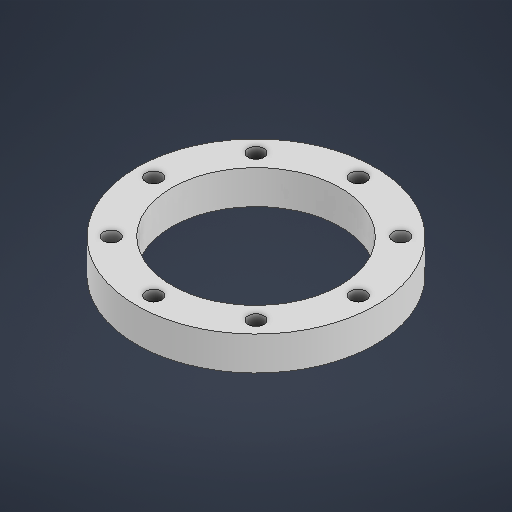
# Autodesk Inventor part: Magnet Spacer
Saved by Autodesk Inventor 2025 (Build 290162000, 162)
## iProperties
Created: 2024-07-10
Part Number: Magnet Spacer
Material: Generic
Document SubType Name: Modeling
Designer: mayhe
Density: 1 g/cm^3
Appearance: Default
Author: mayhe
Autodesk Inventor part; units mm, degrees
ref_plane "YZ Plane" through (0, 0, 0) normal (1, 0, 0) x (0, 1, 0)
ref_plane "XZ Plane" through (0, 0, 0) normal (0, 1, 0) x (-1, 0, 0)
ref_plane "XY Plane" through (0, 0, 0) normal (0, 0, 1) x (1, 0, 0)
sketch "Sketch1" plane through (0, 0, 0) normal (0, 1, 0) x (-1, 0, 0)
  circle A0 centre (0, 0) radius 53.125
  circle A1 centre (0, 0) radius 37.5
  dimension "d0" = 106.25
  dimension "d1" = 75
  constraints: 2 centre point, 2 coincident
  measures "d0" diameter of A0
  measures "d1" diameter of A1
extrude "Extrusion1" add sketch "Sketch1" along normal blind 15
sketch "Sketch2" plane through (0, 0, 0) normal (0, -1, 0) x (1, 0, 0)
  circle A0 centre (0, 0) radius 41.25
  circle A1 centre (-41.25, 0) radius 2.5
  circle A2 centre (-29.1682, -29.1682) radius 2.5
  circle A3 centre (0, -41.25) radius 2.5
  circle A4 centre (29.1682, -29.1682) radius 2.5
  circle A5 centre (41.25, 0) radius 2.5
  circle A6 centre (29.1682, 29.1682) radius 2.5
  circle A7 centre (0, 41.25) radius 2.5
  circle A8 centre (-29.1682, 29.1682) radius 2.5
  dimension "d4" = 82.5
  dimension "d5" = 5
  dimension "d8" = 360
  constraints: 8 centre point, 1 coincident, 1 horizontal alignment, 19 other
  measures "d5" diameter of A1
extrude "Extrusion2" cut sketch "Sketch2" against normal blind 3 contours A0 A5 | A0 A5 | A6 A0 | A0 A6 | A4 A0 | A0 A4 | A7 A0 | A0 A7 | A3 A0 | A0 A3 | A8 A0 | A0 A8 | A2 A0 | A0 A2 | A1 A0 | A0 A1
sketch "Sketch3" plane through (0, 15, 0) normal (0, 1, 0) x (1, 0, 0)
  circle A0 centre (0, 0) radius 45.5
  circle A1 centre (45.5, 0) radius 3.5
  circle A2 centre (32.1734, 32.1734) radius 3.5
  circle A3 centre (0, 45.5) radius 3.5
  circle A4 centre (-32.1734, 32.1734) radius 3.5
  circle A5 centre (-45.5, 0) radius 3.5
  circle A6 centre (-32.1734, -32.1734) radius 3.5
  circle A7 centre (0, -45.5) radius 3.5
  circle A8 centre (32.1734, -32.1734) radius 3.5
  dimension "d12" = 91
  dimension "d13" = 7
  dimension "d16" = 360
  constraints: 8 centre point, 1 coincident, 1 horizontal alignment, 19 other
  measures "d13" diameter of A1
extrude "Extrusion3" cut sketch "Sketch3" against normal blind 7 contours A0 A1 | A0 A1 | A2 A0 | A0 A2 | A8 A0 | A0 A8 | A3 A0 | A0 A3 | A7 A0 | A0 A7 | A4 A0 | A0 A4 | A6 A0 | A0 A6 | A5 A0 | A0 A5
body "Solid1"
